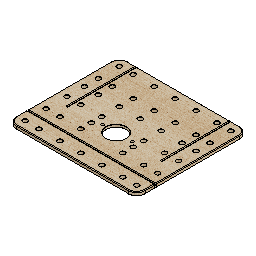
model (Autodesk Fusion 360 design; units mm, degrees)
Autodesk Fusion 360 part; units mm, degrees
note: some values were not read from the file. Set by a fixed rule: which face or edge a step refers to.
sketch "bench" plane through (0, 0, 0) normal (0, 0, 1) x (1, 0, 0)
  line L0 (0, 0) -> (608, 0)
  line L1 (608, 0) -> (608, 448)
  line L2 (608, 448) -> (0, 448)
  line L3 (0, 448) -> (0, 0)
  circle A0 centre (112, 112) radius 10
  circle A1 centre (208, 112) radius 10
  circle A2 centre (304, 112) radius 10
  circle A3 centre (400, 112) radius 10
  circle A4 centre (496, 112) radius 10
  circle A5 centre (112, 208) radius 10
  circle A6 centre (208, 208) radius 10
  circle A7 centre (304, 208) radius 10
  circle A8 centre (400, 208) radius 10
  circle A9 centre (496, 208) radius 10
  circle A10 centre (112, 304) radius 10
  circle A11 centre (208, 304) radius 10
  circle A12 centre (304, 304) radius 10
  circle A13 centre (400, 304) radius 10
  circle A14 centre (496, 304) radius 10
  circle A15 centre (112, 400) radius 10
  circle A16 centre (208, 400) radius 10
  circle A17 centre (304, 400) radius 10
  circle A18 centre (400, 400) radius 10
  circle A19 centre (496, 400) radius 10
  circle A20 centre (560, 400) radius 10
  circle A21 centre (560, 304) radius 10
  circle A22 centre (560, 208) radius 10
  circle A23 centre (560, 112) radius 10
  circle A24 centre (48, 400) radius 10
  circle A25 centre (48, 304) radius 10
  circle A26 centre (48, 208) radius 10
  circle A27 centre (48, 112) radius 10
  circle A28 centre (48, 48) radius 10
  circle A29 centre (112, 48) radius 10
  circle A30 centre (208, 48) radius 10
  circle A31 centre (304, 48) radius 10
  circle A32 centre (400, 48) radius 10
  circle A33 centre (560, 48) radius 10
  circle A34 centre (496, 48) radius 10
  line L4 (48, 48) -> (0, 48) construction
  line L5 (48, 48) -> (48, 0) construction
  line L6 (560, 48) -> (608, 48) construction
  line L7 (48, 400) -> (48, 448) construction
  dimension "d1" = 20
  dimension "d4" = 96
  dimension "d5" = 96
  dimension "d8" = 64
  dimension "d9" = 0
  dimension "d12" = -64
  dimension "d13" = 0
  dimension "d16" = 0
  dimension "d17" = -64
  dimension "d18" = 48
  constraint horizontal L0
  constraint vertical L1
  constraint horizontal L2
  constraint vertical L3
  constraint coincident L0.start L3.end
  constraint coincident A28.centre L4.start
  constraint coincident L3 L4.end
  constraint coincident L0 L5.end
  constraint horizontal L4
  constraint vertical L5
  constraint equal L4 L5
  constraint coincident A33.centre L6.start
  constraint coincident L1 L6.end
  constraint horizontal L6
  constraint equal L4 L6
  constraint coincident A24.centre L7.start
  constraint coincident L2 L7.end
  constraint vertical L7
  constraint equal L5 L7
  measures "d1" diameter of A0
  measures "d18" distance of L0.start L4.end
sketch "table" plane through (0, 0, 0) normal (0, 0, 1) x (1, 0, 0)
  line L0 (10, 246) -> (598, 246)
  line L1 (598, 246) -> (598, -262)
  line L2 (598, -262) -> (10, -262)
  line L3 (10, -262) -> (10, 246)
  line L4 (304, -62.1314) -> (304, -262) construction
  line L5 (304, 246) -> (304, 400) construction
  line L6 (248, -5) -> (360, -5)
  line L7 (48, 208) -> (10, 208) construction
  line L8 (48, 208) -> (48, 246) construction
  arc A0 (48, 246) -> (10, 208) centre (48, 208) ccw
  arc A1 (598, 208) -> (560, 246) centre (560, 208) ccw
  arc A2 (560, -262) -> (598, -224) centre (560, -224) ccw
  arc A3 (10, -224) -> (48, -262) centre (48, -224) ccw
  circle A4 centre (48, 208) radius 10
  circle A5 centre (48, 112) radius 10
  circle A6 centre (112, 112) radius 10
  circle A7 centre (112, 208) radius 10
  circle A8 centre (208, 208) radius 10
  circle A9 centre (208, 112) radius 10
  circle A10 centre (48, 48) radius 10
  circle A11 centre (112, 48) radius 10
  circle A12 centre (208, 48) radius 10
  circle A13 centre (304, 112) radius 10
  circle A14 centre (304, 208) radius 10
  circle A15 centre (304, 48) radius 10
  circle A16 centre (400, 48) radius 10
  circle A17 centre (400, 112) radius 10
  circle A18 centre (400, 208) radius 10
  circle A19 centre (496, 208) radius 10
  circle A20 centre (496, 112) radius 10
  circle A21 centre (496, 48) radius 10
  circle A22 centre (560, 112) radius 10
  circle A23 centre (560, 208) radius 10
  circle A24 centre (560, 48) radius 10
  circle A25 centre (48, 16) radius 10
  circle A26 centre (112, 16) radius 10
  circle A27 centre (208, 16) radius 10
  circle A28 centre (304, 16) radius 10
  circle A29 centre (400, 16) radius 10
  circle A30 centre (496, 16) radius 10
  circle A31 centre (560, 16) radius 10
  circle A32 centre (48, -80) radius 10
  circle A33 centre (112, -80) radius 10
  circle A34 centre (208, -80) radius 10
  circle A35 centre (304, -80) radius 10
  circle A36 centre (400, -80) radius 10
  circle A37 centre (496, -80) radius 10
  circle A38 centre (560, -80) radius 10
  circle A39 centre (48, -176) radius 10
  circle A40 centre (112, -176) radius 10
  circle A41 centre (208, -176) radius 10
  circle A42 centre (304, -176) radius 10
  circle A43 centre (400, -176) radius 10
  circle A44 centre (496, -176) radius 10
  circle A45 centre (560, -176) radius 10
  circle A46 centre (48, -32) radius 10
  circle A47 centre (112, -32) radius 10
  circle A48 centre (208, -32) radius 10
  circle A49 centre (304, -32) radius 10
  circle A50 centre (400, -32) radius 10
  circle A51 centre (496, -32) radius 10
  circle A52 centre (560, -32) radius 10
  circle A53 centre (48, -128) radius 10
  circle A54 centre (112, -128) radius 10
  circle A55 centre (208, -128) radius 10
  circle A56 centre (304, -128) radius 10
  circle A57 centre (400, -128) radius 10
  circle A58 centre (496, -128) radius 10
  circle A59 centre (560, -128) radius 10
  circle A60 centre (48, -224) radius 10
  circle A61 centre (112, -224) radius 10
  circle A62 centre (208, -224) radius 10
  circle A63 centre (304, -224) radius 10
  circle A64 centre (400, -224) radius 10
  circle A65 centre (496, -224) radius 10
  circle A66 centre (560, -224) radius 10
  circle A67 centre (304, -62.1314) radius 46
  line L9 (224, -62.1314) -> (384, -62.1314) construction
  circle A68 centre (377, -62.1314) radius 3.175
  circle A69 centre (377, -62.1314) radius 6.5
  circle A70 centre (241.5, -62.1314) radius 6.5
  circle A71 centre (241.5, -62.1314) radius 3.175
  line L10 (273.2846, -136) -> (334.7154, -136)
  arc A72 (248, -5) -> (273.2846, -136) centre (304, -62.1314) ccw
  arc A73 (334.7154, -136) -> (360, -5) centre (304, -62.1314) ccw
  point P0 (304, -62.1314)
  point P1 (304, 400)
  point P2 (496, 208)
  point P3 (48, 208)
  point P4 (48, 112)
  dimension "d23" = 508
  dimension "d24" = 588
  dimension "d26" = 160
  dimension "d29" = 102
  dimension "d30" = 112
  dimension "d31" = 199.8686
  dimension "d34" = 0
  dimension "d35" = -96
  dimension "d40" = 5
  dimension "d43" = 0
  dimension "d44" = 48
  dimension "d47" = 0
  dimension "d48" = -48
  dimension "d54" = 92
  dimension "d55" = 6.35
  dimension "d56" = 13
  dimension "d57" = 7
  dimension "d58" = 135.5
  dimension "d65" = 131
  dimension "d66" = 17.5
  constraint horizontal L0
  constraint vertical L1
  constraint horizontal L2
  constraint vertical L3
  constraint coincident P0 L4.start
  constraint midpoint L2 L4.end
  constraint vertical L4
  constraint midpoint L0 L5.start
  constraint coincident P1 L5.end
  constraint vertical L5
  constraint horizontal L6
  constraint coincident P3 L7.start
  constraint coincident L3 L7.end
  constraint coincident L0 L8.end
  constraint horizontal L7
  constraint vertical L8
  constraint equal L7 L8
  constraint tangent L0 A0
  constraint tangent L3 A0
  constraint tangent L0 A1
  constraint coincident L1 A1.start
  constraint coincident L0 A1.end
  constraint tangent L1 A2
  constraint coincident L1 A2.end
  constraint coincident L2 A2.start
  constraint tangent L2 A3
  constraint coincident L2 A3.end
  constraint coincident L3 A3.start
  constraint tangent L3 A3
  constraint tangent L2 A2
  constraint tangent L1 A1
  constraint equal A0 A1
  constraint equal A0 A3
  constraint equal A0 A2
  constraint concentric A67 A72
  constraint coincident L9.start A72
  constraint coincident L9.end A72
  constraint horizontal L9
  constraint coincident P0 L9
  constraint coincident L9 A68.centre
  constraint concentric A68 A69
  constraint coincident L9 A70.centre
  constraint concentric A70 A71
  constraint equal A68 A71
  constraint equal A69 A70
  constraint coincident L10.end A72
  constraint horizontal L10
  constraint concentric A72 A73
  measures "d23" distance of L0.start L2.end
  measures "d24" distance of L0.start L0.end
  measures "d26" diameter of A72
  measures "d29" distance of L1 P2
  measures "d30" distance of L6.start L6.end
  measures "d31" distance of P0 L4.end
  measures "d40" vertical distance of L6.start origin
  measures "d54" diameter of A67
  measures "d55" diameter of A68
  measures "d56" diameter of A69
  measures "d57" distance of L9.end A68.centre
  measures "d58" distance of A68.centre A70.centre
  measures "d65" distance of L6 L10
  measures "d66" distance of L9.start A70.centre
extrude "Extrude1" add sketch "table" against normal blind 18 contours L0 L1 L2 L3 A0 A1 A2 A3 | L6 A56 L10 A72 A73 | A56 L10 | A56 L10 | A4 | A5 | A6 | A7 | A8 | A9 | A10 | A11 | A12 | A13 | A14 | A15 | A16 | A17 | A18 | A19 | A20 | A21 | A22 | A23 | A24 | A25 | A26 | A27 | A28 | A29 | A30 | A31 | A32 | A33 | A34 | A35 | A36 | A37 | A38 | A39 | A40 | A41 | A42 | A43 | A44 | A45 | A46 | A47 | A48 | A49 | A50 | A51 | A52 | A53 | A54 | A55 | A57 | A58 | A59 | A60 | A61 | A62 | A63 | A64 | A65 | A66 | A67 | A68 | A69 | A70 | A71
extrude "Extrude2" cut sketch "bench" sketch "table" against normal blind 25 contours A0 | A1 | A2 | A3 | A4 | A5 | A6 | A7 | A8 | A9 | A22 | A23 | A27 | A28 | A29 | A30 | A31 | A32 | A33 | A34 of sketch 2 contours A4 | A34 | A35 | A36 | A46 | A47 | A48 | A49 | A50 | A51 | A52 | A53 | A54 | A55 | A57 | A58 | A59 | A60 | A61 | A62 | A63 | A64 | A65 | A66 | A67 | A68 | A71
extrude "Extrude3" cut sketch "table" against normal blind 6.5 contours A69 | A70
extrude "Extrude4" cut sketch "table" along normal blind 6 from surface at -18 contours L6 A56 L10 A72 A73 | A56 L10 | A69 | A70 picked at (301.9506, -132.2041)
sketch "tape lines" plane through (0, 0, 0) normal (0, 0, 1) x (-1, 0, 0)
  circle A0 centre (-241.5, 62.1314) radius 6.5
  circle A1 centre (-377, 62.1314) radius 6.5
  arc A2 (-48, -246) -> (-10, -208) centre (-48, -208) ccw
  line L0 (-10, -208) -> (-10, 224)
  arc A3 (-10, 224) -> (-48, 262) centre (-48, 224) ccw
  line L1 (-48, 262) -> (-560, 262)
  arc A4 (-560, 262) -> (-598, 224) centre (-560, 224) ccw
  line L2 (-598, 224) -> (-598, -208)
  arc A5 (-598, -208) -> (-560, -246) centre (-560, -208) ccw
  line L3 (-560, -246) -> (-48, -246)
  line L4 (-560, -208) -> (-560, -112) construction
  line L5 (-560, -112) -> (-560, -48) construction
  line L6 (-560, -48) -> (-560, 32) construction
  line L7 (-560, 32) -> (-560, 128) construction
  line L8 (-560, 128) -> (-560, 224) construction
  circle A6 centre (-304, 62.1314) radius 46
  circle A7 centre (-304, 224) radius 10
  circle A8 centre (-560, 128) radius 10
  circle A9 centre (-208, 80) radius 10
  circle A10 centre (-560, 32) radius 10
  circle A11 centre (-112, 32) radius 10
  circle A12 centre (-48, 32) radius 10
  circle A13 centre (-496, 32) radius 10
  circle A14 centre (-208, 128) radius 10
  circle A15 centre (-496, 128) radius 10
  circle A16 centre (-208, 224) radius 10
  circle A17 centre (-560, 224) radius 10
  circle A18 centre (-496, -48) radius 10
  circle A19 centre (-112, -48) radius 10
  circle A20 centre (-400, -112) radius 10
  circle A21 centre (-304, -208) radius 10
  circle A22 centre (-112, -208) radius 10
  circle A23 centre (-560, -208) radius 10
  circle A24 centre (-112, -112) radius 10
  circle A25 centre (-400, -208) radius 10
  circle A26 centre (-304, -112) radius 10
  circle A27 centre (-208, -48) radius 10
  circle A28 centre (-400, -48) radius 10
  circle A29 centre (-48, -112) radius 10
  circle A30 centre (-496, -112) radius 10
  circle A31 centre (-208, -208) radius 10
  circle A32 centre (-560, -48) radius 10
  circle A33 centre (-48, -48) radius 10
  circle A34 centre (-208, -112) radius 10
  circle A35 centre (-496, -208) radius 10
  circle A36 centre (-560, -112) radius 10
  circle A37 centre (-304, -48) radius 10
  circle A38 centre (-400, 224) radius 10
  circle A39 centre (-48, 224) radius 10
  circle A40 centre (-48, 128) radius 10
  circle A41 centre (-400, 80) radius 10
  circle A42 centre (-208, 32) radius 10
  circle A43 centre (-48, -208) radius 10
  circle A44 centre (-400, 32) radius 10
  circle A45 centre (-400, 128) radius 10
  circle A46 centre (-112, 128) radius 10
  circle A47 centre (-112, 224) radius 10
  circle A48 centre (-496, 224) radius 10
  point P0 (-560, 176)
  point P1 (-560, 80)
  point P2 (-560, -8)
  point P3 (-560, -80)
  point P4 (-560, -160)
  dimension "d68" = 86
  dimension "d69" = 182
  dimension "d70" = 270
  dimension "d71" = 342
  dimension "d72" = 422
  constraint coincident A5.centre L4.start
  constraint coincident A4.centre L8.end
  constraint midpoint L8 P0
  constraint midpoint L7 P1
  constraint midpoint L6 P2
  constraint midpoint L5 P3
  constraint midpoint L4 P4
  measures "d68" distance of L1 P0
  measures "d69" distance of L1 P1
  measures "d70" distance of L1 P2
  measures "d71" distance of L1 P3
  measures "d72" distance of L1 P4
chamfer "Chamfer2" distance 1 angle 45 6 edges at (261.1129, -45.4971, 0) (261.1129, -45.4971, -12) (225.4498, -77.2926, -18) (304, -5, -18) (382.5502, -77.2926, -18) (304, -136, -18) 42 faces at (563.1849, 217.4793, -6) (563.1849, 121.4793, -6) (563.1849, 57.4793, -6) (563.1849, -22.5207, -6) (563.1849, -118.5207, -6) (563.1849, -214.5207, -6) (505.9503, 207.0043, -6) (505.9503, 111.0043, -6) (505.9503, 47.0043, -6) (505.9503, -32.9957, -6) (505.9503, -128.9957, -6) (505.9503, -224.9957, -6) (409.9503, 207.0043, -6) (409.9503, 111.0043, -6) (409.9503, 47.0043, -6) (409.9503, -32.9957, -6) (409.9503, -80.9957, -6) (409.9503, -128.9957, -6) (409.9503, -224.9957, -6) (313.9503, 207.0043, -6) (313.9503, 111.0043, -6) (313.9503, 47.0043, -6) (313.9503, -224.9957, -6) (217.9503, 207.0043, -6) (217.9503, 111.0043, -6) (217.9503, 47.0043, -6) (217.9503, -32.9957, -6) (217.9503, -80.9957, -6) (217.9503, -128.9957, -6) (217.9503, -224.9957, -6) (121.9503, -224.9957, -6) (121.9503, -128.9957, -6) (121.9503, -32.9957, -6) (121.9503, 47.0043, -6) (121.9503, 111.0043, -6) (121.9503, 207.0043, -6) (57.9503, 207.0043, -6) (57.9503, 111.0043, -6) (57.9503, 47.0043, -6) (57.9503, -32.9957, -6) (57.9503, -128.9957, -6) (57.9503, -224.9957, -6)
fillet "Fillet1" radius 3.175 16 edges at (21.1299, -250.8701, 0) (10, -8, 0) (21.1299, 234.8701, 0) (304, 246, 0) (586.8701, 234.8701, 0) (598, -8, 0) (586.8701, -250.8701, 0) (304, -262, 0) (10, -8, -18) (21.1299, 234.8701, -18) (304, 246, -18) (586.8701, 234.8701, -18) (598, -8, -18) (586.8701, -250.8701, -18) (304, -262, -18) (21.1299, -250.8701, -18)
sketch "track locations" plane through (0, 0, 0) normal (0, 0, 1) x (-1, 0, 0)
  circle A0 centre (-48, 224) radius 11
  circle A1 centre (-48, 32) radius 11
  circle A2 centre (-48, -112) radius 11
  circle A3 centre (-112, -208) radius 11
  circle A4 centre (-112, -48) radius 11
  circle A5 centre (-112, 128) radius 11
  circle A6 centre (-208, 224) radius 11
  circle A7 centre (-208, 80) radius 11
  circle A8 centre (-208, -48) radius 11
  circle A9 centre (-208, -208) radius 11
  circle A10 centre (-304, -48) radius 11
  circle A11 centre (-304, -208) radius 11
  circle A12 centre (-400, 128) radius 11
  circle A13 centre (-400, 32) radius 11
  circle A14 centre (-400, -112) radius 11
  circle A15 centre (-496, 224) radius 11
  circle A16 centre (-496, 32) radius 11
  circle A17 centre (-496, -112) radius 11
  circle A18 centre (-560, 224) radius 11
  circle A19 centre (-560, 32) radius 11
  circle A20 centre (-560, -112) radius 11
  circle A21 centre (-304, 62.1314) radius 47
  circle A22 centre (-241.5, 62.1314) radius 6.5
  circle A23 centre (-377, 62.1314) radius 6.5
  circle A24 centre (-560, -208) radius 11
  circle A25 centre (-560, -48) radius 11
  circle A26 centre (-560, 128) radius 11
  circle A27 centre (-496, -208) radius 11
  circle A28 centre (-496, -48) radius 11
  circle A29 centre (-496, 128) radius 11
  circle A30 centre (-400, -208) radius 11
  circle A31 centre (-400, -48) radius 11
  circle A32 centre (-400, 80) radius 11
  circle A33 centre (-400, 224) radius 11
  circle A34 centre (-304, -112) radius 11
  circle A35 centre (-304, 224) radius 11
  circle A36 centre (-208, -112) radius 11
  circle A37 centre (-208, 32) radius 11
  circle A38 centre (-208, 128) radius 11
  circle A39 centre (-112, 224) radius 11
  circle A40 centre (-112, 32) radius 11
  circle A41 centre (-112, -112) radius 11
  circle A42 centre (-48, -208) radius 11
  circle A43 centre (-48, -48) radius 11
  circle A44 centre (-48, 128) radius 11
  arc A45 (-13.175, 224) -> (-48, 258.825) centre (-48, 224) ccw
  line L0 (-48, 258.825) -> (-560, 258.825)
  arc A46 (-560, 258.825) -> (-594.825, 224) centre (-560, 224) ccw
  line L1 (-594.825, 224) -> (-594.825, -208)
  arc A47 (-594.825, -208) -> (-560, -242.825) centre (-560, -208) ccw
  line L2 (-560, -242.825) -> (-48, -242.825)
  arc A48 (-48, -242.825) -> (-13.175, -208) centre (-48, -208) ccw
  line L3 (-13.175, -208) -> (-13.175, 224)
  line L4 (-88.1, -246) -> (-88.1, 262)
  line L5 (-519.9, -246) -> (-519.9, 262)
  line L6 (-88.1, 62.1314) -> (-519.9, 62.1314) construction
  line L7 (-10, 176) -> (-598, 176)
  line L8 (-560, 262) -> (-48, 262)
  line L9 (-48, -246) -> (-560, -246)
  line L10 (-10, -208) -> (-10, 224)
  line L11 (-598, 224) -> (-598, -208)
  point P0 (-304, 62.1314)
  dimension "d75" = 431.8
  dimension "d76" = 86
  constraint vertical L4
  constraint vertical L5
  constraint equal L4 L5
  constraint coincident L4 L6.start
  constraint coincident L5 L6.end
  constraint midpoint L6 P0
  constraint horizontal L6
  constraint coincident P0 A21.centre
  constraint horizontal L7
  constraint coincident L7.start L10
  constraint coincident L7.end L11
  constraint coincident L5.end L8
  constraint coincident L5.start L9
  constraint coincident L4.start L9
  measures "d75" horizontal distance of L4.start L5.start
  measures "d76" distance of L7 L8
sketch "featherboard profile" plane through (10, 0, 0) normal (-1, 0, 0) x (0, -1, 0)
  line L0 (-208, -14.825) -> (224, -14.825)
  line L1 (224, -14.825) -> (224, -3.175)
  line L2 (224, -3.175) -> (-208, -3.175)
  line L3 (-208, -3.175) -> (-208, -14.825)
  line L4 (172, 0) -> (180, 0)
  line L5 (172, 0) -> (172, -6.5)
  line L6 (172, -6.5) -> (169.75, -6.5)
  line L7 (169.75, -6.5) -> (169.75, -12.75)
  line L8 (169.75, -12.75) -> (182.25, -12.75)
  line L9 (182.25, -12.75) -> (182.25, -6.5)
  line L10 (182.25, -6.5) -> (180, -6.5)
  line L11 (180, -6.5) -> (180, 0)
  point P0 (176, 0)
  dimension "d77" = 8
  dimension "d78" = 6.5
  dimension "d79" = 12.75
  dimension "d80" = 12.5
  constraint horizontal L4
  constraint midpoint P0 L4
  constraint vertical L7
  constraint horizontal L6
  constraint vertical L5
  constraint vertical L9
  constraint horizontal L10
  constraint vertical L11
  constraint horizontal L8
  constraint equal L5 L11
  constraint equal L6 L10
  measures "d77" distance of L5 L11
  measures "d78" distance of L4 L6
  measures "d79" distance of L4 L8
  measures "d80" distance of L6.end L9.end
sweep "Sweep1" cut profiles "featherboard profile" path "track locations" along L7 section 1 contours L2 L4 L5 L11 | L2 L5 L6 L7 L8 L9 L10 L11
sketch "fence profile" plane through (0, -262, 0) normal (0, -1, 0) x (1, 0, 0)
  line L0 (48, -14.825) -> (560, -14.825)
  line L1 (560, -14.825) -> (560, -3.175)
  line L2 (560, -3.175) -> (48, -3.175)
  line L3 (48, -3.175) -> (48, -14.825)
  line L4 (84.1, 0) -> (92.1, 0)
  line L5 (84.1, 0) -> (84.1, -6.5)
  line L6 (84.1, -6.5) -> (81.725, -6.5)
  line L7 (81.725, -6.5) -> (81.725, -12.75)
  line L8 (81.725, -12.75) -> (94.475, -12.75)
  line L9 (94.475, -12.75) -> (94.475, -6.5)
  line L10 (94.475, -6.5) -> (92.1, -6.5)
  line L11 (92.1, -6.5) -> (92.1, 0)
  line L12 (526.275, -6.5) -> (523.9, -6.5)
  line L13 (523.9, -6.5) -> (523.9, 0)
  line L14 (515.9, 0) -> (523.9, 0)
  line L15 (515.9, 0) -> (515.9, -6.5)
  line L16 (515.9, -6.5) -> (513.525, -6.5)
  line L17 (513.525, -6.5) -> (513.525, -12.75)
  line L18 (526.275, -12.75) -> (526.275, -6.5)
  line L19 (513.525, -12.75) -> (526.275, -12.75)
  point P0 (88.1, 0)
  point P1 (519.9, 0)
  dimension "d87" = 431.8
  dimension "d88" = 8
  dimension "d89" = 12.75
  dimension "d90" = 12.75
  dimension "d93" = 431.8
  dimension "d94" = 0
  dimension "d101" = 6.5
  constraint horizontal L4
  constraint midpoint P0 L4
  constraint horizontal L8
  constraint horizontal L6
  constraint vertical L7
  constraint vertical L5
  constraint vertical L11
  constraint horizontal L10
  constraint vertical L9
  constraint equal L7 L9
  constraint equal L6 L10
  measures "d87" distance of P0 P1
  measures "d88" distance of L4.start L4.end
  measures "d89" vertical distance of L4.start L7.end
  measures "d90" distance of L6.end L9.end
  measures "d101" vertical distance of L4.start L6.end
extrude "Extrude5" cut sketch "fence profile" against normal up to surface (318 mm away) from surface at -190 contours L2 L4 L5 L11 | L2 L5 L6 L7 L8 L9 L10 L11 | L2 L12 L13 L15 L16 L17 L18 L19 | L2 L13 L14 L15
equation "maxA = 608 mm - margin - 5 mm"
equation "maxB = 523 mm - margin"
equation "d23 = maxB"
equation "d24 = maxA"
equation "margin = 15 mm"
equation "d74 = 1/8\""
equation "d75 = 17\""
equation "d88 = d77"
equation "d89 = d79"
equation "d90 = d89"
equation "d93 = d87"
equation "d101 = d78"
